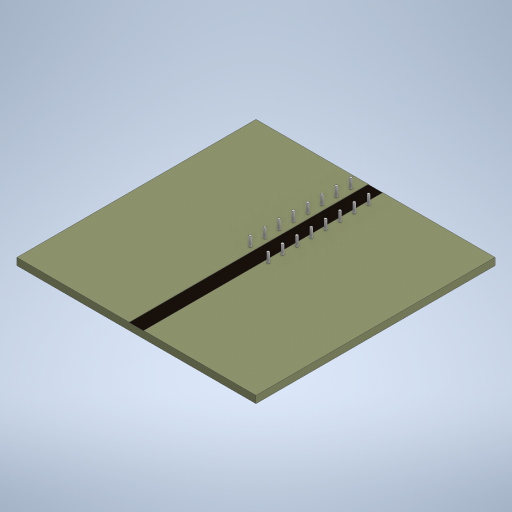
# Autodesk Inventor part: forest
Saved by Autodesk Inventor 2023 (Build 270158000, 158)
## iProperties
Created: 2022-11-04
Part Number: forest
Material: Generic
Document SubType Name: Modeling
Designer: derm
Density: 1 g/cm^3
Appearance: Default
Author: derm
Autodesk Inventor part; units mm, degrees
ref_plane "YZ Plane" through (0, 0, 0) normal (1, 0, 0) x (0, 1, 0)
ref_plane "XZ Plane" through (0, 0, 0) normal (0, 1, 0) x (-1, 0, 0)
ref_plane "XY Plane" through (0, 0, 0) normal (0, 0, 1) x (1, 0, 0)
sketch "Sketch1" plane through (0, 0, 0) normal (0, 1, 0) x (-1, 0, 0)
  line L0 (-50000, 50000) -> (50000, 50000)
  line L1 (50000, 50000) -> (50000, -50000)
  line L2 (50000, -50000) -> (-50000, -50000)
  line L3 (-50000, -50000) -> (-50000, 50000)
  line L4 (-50000, 50000) -> (50000, -50000) construction
  line L5 (50000, 50000) -> (-50000, -50000) construction
  point P0 (0, 0)
  dimension "d0" = 100000
  dimension "d1" = 100000
  constraints: 12 end point, 2 midpoint, 2 parallel, 1 horizontal, 1 perpendicular
  measures "d0" distance of L0.end L1.end
  measures "d1" distance of L1.end L2.end
extrude "Extrusion1" add sketch "Sketch1" against normal blind 3000
sketch "Sketch2" plane through (0, 0, 0) normal (0, 1, 0) x (1, 0, 0)
  line L0 (-50000, 50000) -> (50000, 50000) projected
  line L1 (3000, -50000) -> (-3000, -50000)
  line L2 (-3000, -50000) -> (-3000, 50000)
  line L3 (-3000, 50000) -> (3000, 50000)
  line L4 (3000, 50000) -> (3000, -50000)
  line L5 (3000, -50000) -> (-3000, 50000) construction
  line L6 (-3000, -50000) -> (3000, 50000) construction
  point P0 (0, 0)
  dimension "d4" = 6000
  constraints: 12 end point, 2 midpoint, 2 parallel, 1 horizontal, 1 perpendicular, 1 point on line
  measures "d4" distance between parallel lines of L4 L2
extrude "Extrusion2" cut sketch "Sketch2" against normal blind 100
sketch "Sketch3" plane through (0, 0, 0) normal (0, 1, 0) x (1, 0, 0)
  line L0 (3000, 50000) -> (3000, -50000) projected
  line L1 (3000, -50000) -> (50000, -50000) projected
  line L2 (50000, -50000) -> (50000, 50000) projected
  line L3 (50000, 50000) -> (3000, 50000) projected
  circle A0 centre (-5162.0769, 2791.8732) radius 500
  circle A1 centre (4518.6624, 580.7791) radius 500
  point P0 (0, 0)
  dimension "d7" = 1000
  dimension "d8" = 1000
  constraints: 2 centre point
  measures "d7" diameter of A0
  measures "d8" diameter of A1
extrude "Extrusion3" add sketch "Sketch3" along normal blind 4000 contours A0 | A1
pattern_linear "Rectangular Pattern1" count 8 spacing 6000 along (0, 0, -1) of "Extrusion3"
body "Solid1"
